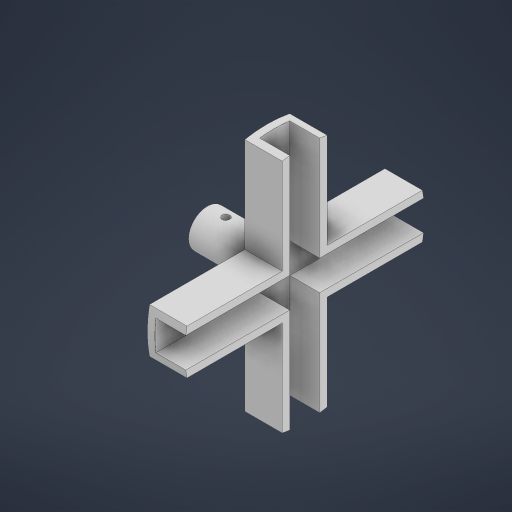
# Autodesk Inventor part: Cross
Saved by Autodesk Inventor 2023.2 (Build 272271000, 271)
## iProperties
Created: 2023-01-16
Part Number: Cross
Material: Generic
Document SubType Name: Modeling
Designer: iusti
Density: 1 g/cm^3
Appearance: Default
Author: iusti
Autodesk Inventor part; units mm, degrees
ref_plane "YZ Plane" through (0, 0, 0) normal (1, 0, 0) x (0, 1, 0)
ref_plane "XZ Plane" through (0, 0, 0) normal (0, 1, 0) x (-1, 0, 0)
ref_plane "XY Plane" through (0, 0, 0) normal (0, 0, 1) x (1, 0, 0)
sketch "Sketch1" plane through (0, 0, 0) normal (1, 0, 0) x (0, 1, 0)
  circle A0 centre (0, 0) radius 32
  dimension "d0" = 64
  constraints: 1 centre point, 1 coincident
  measures "d0" diameter of A0
extrude "Extrusion1" add sketch "Sketch1" along normal blind 10
sketch "Sketch2" plane through (10, 0, 0) normal (1, 0, 0) x (0, 0, -1)
  circle A0 centre (0, 0) radius 32 projected
  line L0 (-6, 33.1057) -> (-6, 6)
  line L1 (-6, 6) -> (-33.1057, 6)
  line L2 (0, 0) -> (-11.4167, 0)
  line L3 (0, 0) -> (0, 10.4167)
  arc A1 (-6, 33.1057) -> (-33.1057, 6) centre (-1.4332, 1.4332) ccw
  line L4 (-6, -33.1057) -> (-6, -6)
  line L5 (-6, -6) -> (-33.1057, -6)
  arc A2 (-33.1057, -6) -> (-6, -33.1057) centre (-1.4332, -1.4332) ccw
  line L6 (6, 33.1057) -> (6, 6)
  line L7 (6, 6) -> (33.1057, 6)
  arc A3 (33.1057, 6) -> (6, 33.1057) centre (1.4332, 1.4332) ccw
  arc A4 (6, -33.1057) -> (33.1057, -6) centre (1.4332, -1.4332) ccw
  line L8 (6, -33.1057) -> (6, -6)
  line L9 (6, -6) -> (33.1057, -6)
  dimension "d3" = 12
  dimension "d4" = 12
  constraints: 20 end point, 12 symmetric about line, 8 point on circle, 4 centre point, 2 perpendicular, 2 vertical, 1 equal radius, 1 horizontal, 3 other
  measures "d3" diameter of L1 L2
  measures "d4" diameter of L0 L3
extrude "Extrusion2" cut sketch "Sketch2" against normal blind 10 contours L7 L6 A0 | A0 L6 A3 L7 | L9 A4 L8 A0 | A0 L8 L9 | L0 L1 A0 | A0 L1 A1 L0 | L4 A2 L5 A0 | A0 L5 L4
shell "Shell1" thickness 2 removed faces 5 at (6.6667, 31.8245, -3.347) at (10, -0.6702, -14.6456) at (6.6667, 0.6706, -31.993) at (6.6667, -31.993, -0.6706) at (6.6667, -0.6706, 31.993)
sketch "Sketch3" plane through (0, 0, 0) normal (-1, 0, 0) x (0, 0, 1)
  arc A0 (-31.4325, 6) -> (-31.4325, -6) centre (0, 0) ccw projected
  circle A1 centre (0, 0) radius 5
  dimension "d9" = 10
  constraints: 1 centre point, 1 coincident
  measures "d9" diameter of A1
extrude "Extrusion3" add sketch "Sketch3" along normal blind 16
sketch "Sketch4" plane through (0, 0, 0) normal (0, 1, 0) x (-1, 0, 0)
  circle A0 centre (11, 0) radius 1
  line L0 (16, -5) -> (16, 5) projected
  point P0 (0, 0)
  dimension "d12" = 2
  dimension "d13" = 5
  constraints: 1 centre point
  measures "d12" diameter of A0
  measures "d13" distance from line of L0 A0.centre
extrude "Extrusion4" cut sketch "Sketch4" along normal mid plane 16
body "Solid1"
